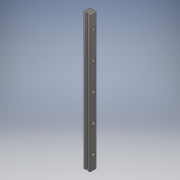
# Autodesk Inventor part: Linearführung
Saved by Autodesk Inventor 2019 (Build 230136000, 136)
## iProperties
Created: 2021-04-25
Part Number: Linearführung
Material: Edelstahl
Document SubType Name: Modeling
Designer: Michael Sumper
Density: 8 g/cm^3
Appearance: Halbpoliert
Author: Michael Sumper
Autodesk Inventor part; units mm, degrees
ref_plane "YZ Plane" through (0, 0, 0) normal (1, 0, 0) x (0, 1, 0)
ref_plane "XZ Plane" through (0, 0, 0) normal (0, 1, 0) x (-1, 0, 0)
ref_plane "XY Plane" through (0, 0, 0) normal (0, 0, 1) x (1, 0, 0)
sketch "Skizze1" plane through (0, 0, 0) normal (0, 1, 0) x (-1, 0, 0)
  line L0 (0, 0) -> (0, -15)
  line L1 (0, -15) -> (5, -15)
  line L2 (5, -15) -> (10, -15) construction
  line L3 (10, -15) -> (15, -15)
  line L4 (15, -15) -> (15, 0)
  line L5 (15, 0) -> (10, 0)
  line L6 (10, 0) -> (5, 0) construction
  line L7 (5, 0) -> (0, 0)
  line L8 (0, -7.5) -> (0, -5.25) construction
  line L9 (0, -5.25) -> (0, -9.75) construction
  line L10 (0, -9.75) -> (9.7, -9.75) construction
  line L11 (0, -5.25) -> (9.7, -5.25) construction
  line L12 (15, -7.5) -> (15, -3.9) construction
  line L13 (15, -3.9) -> (15, -11.4) construction
  line L14 (15, -11.4) -> (9.7, -11.4) construction
  line L15 (9.7, -11.4) -> (9.7, -9.75) construction
  line L16 (15, -3.9) -> (9.7, -3.9) construction
  line L17 (9.7, -3.9) -> (9.7, -5.25) construction
  line L18 (10, 0) -> (8.5, -2.5981)
  line L19 (10, 0) -> (13, 0) construction
  line L20 (5, 0) -> (6.5, -2.5981)
  line L21 (5, 0) -> (8, 0) construction
  line L22 (6.5, -2.5981) -> (8.5, -2.5981)
  line L23 (10, -15) -> (8.5, -12.4019)
  line L24 (10, -15) -> (13, -15) construction
  line L25 (5, -15) -> (6.5, -12.4019)
  line L26 (5, -15) -> (8, -15) construction
  line L27 (6.5, -12.4019) -> (8.5, -12.4019)
  dimension "d0" = 15
  dimension "d1" = 5
  dimension "d2" = 5
  dimension "d3" = 5
  dimension "d4" = 15
  dimension "d5" = 5
  dimension "d6" = 5
  dimension "d7" = 2.25
  dimension "d8" = 4.5
  dimension "d9" = 9.7
  dimension "d10" = 9.7
  dimension "d11" = 3.6
  dimension "d12" = 7.5
  dimension "d13" = 5.3
  dimension "d14" = 3
  dimension "d15" = 120
  dimension "d16" = 3
  dimension "d17" = 60
  dimension "d18" = 3
  dimension "d19" = 120
  dimension "d20" = 3
  dimension "d21" = 60
  constraints: 56 end point, 7 horizontal, 6 perpendicular, 6 point on line, 4 equal length, 2 midpoint, 1 parallel, 1 vertical
  measures "d0" distance of L0.start L0.end
  measures "d1" distance of L0.end L1.end
  measures "d2" distance of L1.end L2.end
  measures "d3" distance of L2.end L3.end
  measures "d4" distance of L3.end L4.end
  measures "d5" distance of L4.end L5.end
  measures "d6" distance of L5.end L6.end
  measures "d7" distance of L8.start L8.end
  measures "d8" distance of L8.end L9.end
  measures "d9" distance of L9.end L10.end
  measures "d10" distance of L8.end L11.end
  measures "d11" distance of L12.start L12.end
  measures "d12" distance of L12.end L13.end
  measures "d13" distance of L13.end L14.end
  measures "d14" distance of L5.end L18.end
  measures "d15" angle of L18 L19
  measures "d16" distance of L6.end L20.end
  measures "d17" angle of L20 L21
  measures "d18" distance of L2.end L23.end
  measures "d19" angle of L24 L23
  measures "d20" distance of L1.end L25.end
  measures "d21" angle of L26 L25
extrude "Extrusion1" add sketch "Skizze1" along normal blind 300
sketch "Skizze2" plane through (0, 0, 0) normal (1, 0, 0) x (0, 0, -1)
  line L0 (15, 300) -> (0, 300) construction
  line L1 (7.5, 300) -> (7.5, 270) construction
  line L2 (7.5, 270) -> (7.5, 210) construction
  line L3 (7.5, 210) -> (7.5, 150) construction
  line L4 (7.5, 150) -> (7.5, 90) construction
  line L5 (7.5, 90) -> (7.5, 30) construction
  point P0 (0, 0)
  dimension "d25" = 30
  dimension "d26" = 60
  dimension "d27" = 60
  dimension "d28" = 60
  dimension "d29" = 60
  constraints: 10 end point, 4 point on line, 1 midpoint, 1 vertical
  measures "d25" distance of L1.start L1.end
  measures "d26" distance of L1.end L2.end
  measures "d27" distance of L2.end L3.end
  measures "d28" distance of L3.end L4.end
  measures "d29" distance of L4.end L5.end
hole "Bohrung1" at (0, 270, -7.5) at (0, 210, -7.5) at (0, 150, -7.5) at (0, 90, -7.5) at (0, 30, -7.5) direction (-1, 0, 0) diameter 4.5 end through all counterbore diameter 7.5 counterbore depth 5.3 clearance for "Innensechskantkopfschraube" size "M4" standard "ANSI Metrisches M Profil"
chamfer "Fase1" distance 1 angle 45 4 edges at (0, 150, -15) (0, 150, 0) (-15, 150, -15) (-15, 150, 0)
chamfer "Fase2" distance 0.1 angle 45 5 edges at (0, 270, -3.75) (0, 210, -3.75) (0, 150, -3.75) (0, 90, -3.75) (0, 30, -3.75)
